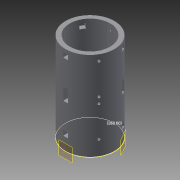
# Autodesk Inventor part: 知能ロボコン外筒改
Saved by Autodesk Inventor 2013 (Build 170138000, 138)
## iProperties
Created: 2014-05-28
Part Number: 知能ロボコン外筒改
Material: 一般
Document SubType Name: Modeling
Designer: horumo136
Density: 1 g/cm^3
Author: horumo136
Autodesk Inventor part; units mm, degrees
ref_plane "YZ Plane" through (0, 0, 0) normal (1, 0, 0) x (0, 1, 0)
ref_plane "XZ Plane" through (0, 0, 0) normal (0, 1, 0) x (-1, 0, 0)
ref_plane "XY Plane" through (0, 0, 0) normal (0, 0, 1) x (1, 0, 0)
sketch "スケッチ1" plane through (0, 0, 0) normal (0, 0, 1) x (1, 0, 0)
  circle A0 centre (0, 0) radius 13
  line L0 (0, 13) -> (0, 33)
  circle A1 centre (0, 0) radius 33
  circle A2 centre (0, 0) radius 40
  dimension "d0" = 26
  dimension "d2" = 20
  dimension "d3" = 80
  constraints: 3 coincident, 2 end point, 2 vertical alignment, 1 centre point, 1 vertical, 4 other
  measures "d2" distance of L0.start L0.end
  measures "d3" diameter of A2
extrude "押し出し1" add sketch "スケッチ1" along normal blind 145 contours A2
sketch "スケッチ2" plane through (0, 0, 0) normal (0, 0, -1) x (-1, 0, 0)
  circle A0 centre (0, 0) radius 33 projected
  circle A1 centre (0, 0) radius 40 projected
  line L0 (5.4, 32.5552) -> (-5.4, 32.5552)
  line L1 (0, 0) -> (-10.5703, 0)
  arc A2 (5.4, 32.5552) -> (-5.4, 32.5552) centre (0, 0) ccw
  line L2 (-5.4, 32.5552) -> (5.4, 32.5552)
  line L3 (5.4, 32.5552) -> (5.4, 32.5552)
  line L4 (5.4, 32.5552) -> (-5.4, 32.5552)
  line L5 (-5.4, 32.5552) -> (-5.4, 32.5552)
  line L6 (-5.4, 32.5552) -> (5.4, 32.5552)
  line L7 (5.4, 32.5552) -> (5.4, 33)
  line L8 (5.4, 33) -> (-5.4, 33)
  line L9 (-5.4, 33) -> (-5.4, 32.5552)
  line L10 (-30.8936, -11.6011) -> (-25.4936, -20.9541)
  line L11 (-30.8936, -11.6011) -> (-31.2788, -11.8235)
  line L12 (-31.2788, -11.8235) -> (-25.8788, -21.1765)
  line L13 (-25.8788, -21.1765) -> (-25.4936, -20.9541)
  line L14 (25.4936, -20.9541) -> (30.8936, -11.6011)
  line L15 (25.4936, -20.9541) -> (25.8788, -21.1765)
  line L16 (25.8788, -21.1765) -> (31.2788, -11.8235)
  line L17 (31.2788, -11.8235) -> (30.8936, -11.6011)
  line L18 (-30.8936, -11.6011) -> (-31.2788, -11.8235)
  line L19 (-31.2788, -11.8235) -> (-25.8788, -21.1765)
  line L20 (-25.8788, -21.1765) -> (-25.4936, -20.9541)
  line L21 (-25.4936, -20.9541) -> (-30.8936, -11.6011)
  line L22 (25.4936, -20.9541) -> (25.8788, -21.1765)
  line L23 (25.8788, -21.1765) -> (31.2788, -11.8235)
  line L24 (31.2788, -11.8235) -> (30.8936, -11.6011)
  line L25 (30.8936, -11.6011) -> (25.4936, -20.9541)
  dimension "d6" = 10.8
  dimension "d8" = 10.8
  dimension "d13" = 360
  constraints: 52 end point, 8 parallel, 6 perpendicular, 5 point on circle, 3 horizontal, 1 centre point, 1 collinear, 1 concentric, 31 other
  measures "d6" distance of L0.start L0.end
  measures "d8" distance of L4.end L3.end
extrude "押し出し2" cut sketch "スケッチ2" against normal blind 145 contours L0 A0 | A0 L8 L7 | L17 L16 A0 | A0 L14 | A0 L9 L8 | L16 L15 A0 | L10 A0 | A0 L12 L11 | L13 L12 A0
sketch "スケッチ3" plane through (-5.4, 33, 0) normal (0, -1, 0) x (1, 0, 0)
  line L0 (10.8, 0) -> (10.8, 145) projected
  line L1 (5.4, 0) -> (5.4, 19.5)
  line L2 (5.4, 19.5) -> (5.4, 24.2)
  line L3 (5.4, 24.2) -> (5.4, 74.8)
  circle A0 centre (5.4, 24.2) radius 1.5
  circle A1 centre (5.4, 74.8) radius 1.5
  line L4 (5.4, 74.8) -> (5.4, 79.9)
  line L5 (5.4, 79.9) -> (5.4, 84.6)
  circle A2 centre (5.4, 84.6) radius 1.5
  line L6 (5.4, 84.6) -> (5.4, 135.2)
  circle A3 centre (5.4, 135.2) radius 1.5
  dimension "d15" = 19.5
  dimension "d16" = 4.7
  dimension "d17" = 50.6
  dimension "d18" = 3
  dimension "d19" = 3
  dimension "d20" = 5.1
  dimension "d21" = 4.7
  dimension "d22" = 3
  dimension "d23" = 50.6
  dimension "d24" = 3
  constraints: 12 end point, 5 collinear, 4 centre point, 4 coincident, 1 parallel
  measures "d15" distance of L1.start L1.end
  measures "d16" distance of L1.end L2.end
  measures "d17" distance of L2.end L3.end
  measures "d18" diameter of A0
  measures "d19" diameter of A1
  measures "d20" distance of L4.start L4.end
  measures "d21" distance of L4.end L5.end
  measures "d22" diameter of A2
  measures "d23" distance of L6.start L6.end
  measures "d24" diameter of A3
hole "穴1" at (0, 33, 24.2) at (0, 33, 74.8) at (0, 33, 84.6) at (0, 33, 135.2) direction (0, 1, 0) diameter 3 depth 8 tip angle 118
pattern_circular "円形状パターン1" count 6 over 360 about axis through (0, 0, 0) along (0, 0, 1) of "穴1"
sketch "スケッチ4" plane through (0, 0, 0) normal (0, 0, -1) x (-1, 0, 0)
  circle A0 centre (0, 0) radius 40 projected
  line L0 (30.8936, -11.6011) -> (31.2788, -11.8235) projected
  line L1 (31.2788, -11.8235) -> (25.8788, -21.1765) projected
  line L2 (25.8788, -21.1765) -> (25.4936, -20.9541) projected
  arc A1 (-25.4936, -20.9541) -> (25.4936, -20.9541) centre (0, 0) ccw projected
  line L3 (-25.4936, -20.9541) -> (-25.8788, -21.1765) projected
  line L4 (-25.8788, -21.1765) -> (-31.2788, -11.8235) projected
  line L5 (-31.2788, -11.8235) -> (-30.8936, -11.6011) projected
  arc A2 (-5.4, 32.5552) -> (-30.8936, -11.6011) centre (0, 0) ccw projected
  line L6 (-5.4, 32.5552) -> (-5.4, 33) projected
  line L7 (-5.4, 33) -> (5.4, 33) projected
  line L8 (5.4, 33) -> (5.4, 32.5552) projected
  arc A3 (30.8936, -11.6011) -> (5.4, 32.5552) centre (0, 0) ccw projected
  point P0 (0, 40)
  point P1 (-34.641, 20)
  point P2 (-34.641, -20)
  point P3 (0, -40)
  point P4 (34.641, -20)
  point P5 (34.641, 20)
  dimension "d37" = 360
  constraints: 1 coincident, 1 vertical alignment, 8 other
ref_plane "作業平面1" through (-34.641, 20, 0) normal (-0.8660254, 0.5, 0) x (-0.5, -0.8660254, 0)
ref_plane "作業平面3" through (0, -40, 0) normal (0, -1, 0) x (1, 0, 0)
ref_plane "作業平面7" through (34.641, 20, 0) normal (0.8660254, 0.5, 0) x (-0.5, 0.8660254, 0)
sketch "スケッチ5" plane through (-34.641, 20, 0) normal (-0.8660254, 0.5, 0) x (-0.5, -0.8660254, 0)
  line L0 (0, 0) -> (0, 24.2)
  line L1 (0, 24.2) -> (0, 74.8)
  line L2 (0, 74.8) -> (0, 79.9)
  line L3 (0, 79.9) -> (0, 84.6)
  line L4 (0, 84.6) -> (0, 135.2)
  line L5 (-4, 139.2) -> (4, 139.2)
  line L6 (4, 139.2) -> (4, 131.2)
  line L7 (4, 131.2) -> (-4, 131.2)
  line L8 (-4, 131.2) -> (-4, 139.2)
  line L9 (-4, 139.2) -> (4, 131.2) construction
  line L10 (4, 139.2) -> (-4, 131.2) construction
  line L11 (-4, 89.6) -> (4, 89.6)
  line L12 (4, 89.6) -> (4, 79.6)
  line L13 (4, 79.6) -> (-4, 79.6)
  line L14 (-4, 79.6) -> (-4, 89.6)
  line L15 (-4, 89.6) -> (4, 79.6) construction
  line L16 (4, 89.6) -> (-4, 79.6) construction
  line L17 (-4, 79.8) -> (4, 79.8)
  line L18 (4, 79.8) -> (4, 69.8)
  line L19 (4, 69.8) -> (-4, 69.8)
  line L20 (-4, 69.8) -> (-4, 79.8)
  line L21 (-4, 79.8) -> (4, 69.8) construction
  line L22 (4, 79.8) -> (-4, 69.8) construction
  line L23 (-4, 28.2) -> (4, 28.2)
  line L24 (4, 28.2) -> (4, 20.2)
  line L25 (4, 20.2) -> (-4, 20.2)
  line L26 (-4, 20.2) -> (-4, 28.2)
  line L27 (-4, 28.2) -> (4, 20.2) construction
  line L28 (4, 28.2) -> (-4, 20.2) construction
  dimension "d39" = 24.2
  dimension "d40" = 50.6
  dimension "d41" = 5.1
  dimension "d42" = 4.7
  dimension "d43" = 50.6
  dimension "d44" = 8
  dimension "d45" = 8
  dimension "d46" = 8
  dimension "d47" = 10
  dimension "d48" = 8
  dimension "d49" = 10
  dimension "d50" = 8
  dimension "d51" = 8
  constraints: 58 end point, 8 midpoint, 8 parallel, 4 horizontal, 4 perpendicular, 3 collinear, 1 point on line, 1 vertical
  measures "d39" distance of L0.start L0.end
  measures "d40" distance of L0.end L1.end
  measures "d41" distance of L1.end L2.end
  measures "d42" distance of L2.end L3.end
  measures "d43" distance of L3.end L4.end
  measures "d44" distance of L6.end L7.end
  measures "d45" distance of L5.end L6.end
  measures "d46" distance of L12.end L13.end
  measures "d47" distance of L11.end L12.end
  measures "d48" distance of L18.end L19.end
  measures "d49" distance of L17.end L18.end
  measures "d50" distance of L24.end L25.end
  measures "d51" distance of L23.end L24.end
extrude "押し出し3" cut sketch "スケッチ5" against normal blind 10
pattern_circular "円形状パターン2" count 3 over 360 about axis through (0, 0, 0) along (0, 0, 1) of "押し出し3"
ref_plane "作業平面8" through (0, 40, 0) normal (0, 1, 0) x (-1, 0, 0)
sketch "スケッチ6" plane through (0, 40, 0) normal (0, 1, 0) x (-1, 0, 0)
  line L0 (0, 0) -> (0, 24.2)
  line L1 (0, 24.2) -> (0, 74.8)
  line L2 (0, 74.8) -> (0, 84.6)
  line L3 (0, 84.6) -> (0, 135.2)
  dimension "d57" = 24.2
  dimension "d58" = 50.6
  dimension "d59" = 9.8
  dimension "d60" = 50.6
  constraints: 8 end point, 4 coincident, 3 collinear, 1 vertical
  measures "d57" distance of L0.start L0.end
  measures "d58" distance of L0.end L1.end
  measures "d59" distance of L1.end L2.end
  measures "d60" distance of L2.end L3.end
hole "穴2" at (0, 40, 74.8) at (0, 40, 24.2) at (0, 40, 84.6) at (0, 40, 135.2) direction (0, -1, 0) diameter 3 depth 8 tip angle 118 counterbore diameter 4 counterbore depth 2
pattern_circular "円形状パターン3" count 3 over 360 about axis through (0, 0, 0) along (0, 0, 1) of "穴2"
